Autodesk Inventor part; units mm, degrees
(part 2 of 2)
  dimension "d182" = 8
  dimension "d185" = 360
  dimension "d189" = 10
  dimension "d190" = 0
  dimension "d191" = 20
  dimension "d192" = 40
  dimension "d193" = 3.1
  dimension "d196" = 50
  dimension "d199" = 50
  dimension "d202" = 22
  dimension "d203" = 10
  dimension "d204" = 2
  constraints: 168 end point, 45 centre point, 24 point on circle, 20 tangent, 17 point on line, 12 midpoint, 11 symmetric about line, 10 horizontal, 9 parallel, 6 equal radius, 6 vertical, 4 perpendicular, 1 collinear, 162 other
  measures "d160" distance of L2.end L6.start
  measures "d163" distance of L2.end L14.start
  measures "d166" distance of L28.end L27.end
  measures "d167" distance of L27.end L26.end
  measures "d168" distance from line of L5 point (25, -12)
  measures "d169" distance from line of L4 point (28.5, -7)
  measures "d172" distance of L27.end L32.start
  measures "d175" distance of L27.end L40.start
  measures "d178" diameter of A3
  measures "d179" distance edge to line of A0 L54
  measures "d182" diameter of A6
  measures "d189" radius of A14
  measures "d190" distance between parallel lines of L194 L195
  measures "d191" distance of L196.start L196.end
  measures "d192" distance of L198.end L196.start
  measures "d193" diameter of A156
  measures "d196" distance of A156.centre A157.centre
  measures "d199" distance of A156.centre A161.centre
  measures "d202" distance of L352.end L353.end
  measures "d203" distance of L353.start L352.end
  measures "d204" radius of A206
extrude "Выдавливание10" cut sketch "Эскиз16" against normal blind 10 contours L29 L28 L27 L26 | L35 L34 L33 L32 | L39 L38 L37 L36 | L43 L42 L41 L40 | L47 L46 L45 L44 | L51 L50 L49 L48 | A2 L54 A3 L53 | L56 A5 L57 A4 | A6 | A7 | A8 | A9 | A10 | A11 | A12 | A13 | L199 L198 A158 L197 L196 | A158 L198 L197 | L197 L198 A158 | L200 L201 A166 L202 L203 | A166 L201 | L201 A166 | A156 | A157 | A159 | A160 | A161 | A171 | A176 | L348 A207 L349 A206 L350 A209 L351 A208
